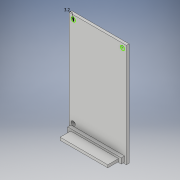
# Autodesk Inventor part: lcd display
Saved by Autodesk Inventor 2017 (Build 210142000, 142)
## iProperties
Created: 2016-11-05
Part Number: lcd display
Material: Generic
Document SubType Name: Modeling
Designer: radrajith
Density: 1 g/cm^3
Appearance: Default
Author: radrajith
Autodesk Inventor part; units mm, degrees
ref_plane "YZ Plane" through (0, 0, 0) normal (1, 0, 0) x (0, 1, 0)
ref_plane "XZ Plane" through (0, 0, 0) normal (0, 1, 0) x (-1, 0, 0)
ref_plane "XY Plane" through (0, 0, 0) normal (0, 0, 1) x (1, 0, 0)
sketch "Sketch1" plane through (0, 0, 0) normal (0, 0, 1) x (1, 0, 0)
  line L0 (42.72, 0) -> (42.72, 77.18)
  line L1 (42.72, 77.18) -> (0, 77.18)
  line L2 (0, 77.18) -> (0, 0)
  line L3 (0, 0) -> (42.72, 0)
  point P0 (0, 0)
  dimension "d0" = 77.18
  dimension "d1" = 42.72
  constraints: 8 end point, 2 parallel, 1 perpendicular
  measures "d0" distance of L2.end L1.end
  measures "d1" distance of L1.end L0.end
extrude "Extrusion1" add sketch "Sketch1" along normal blind 2
sketch "Sketch3" plane through (0, 0, 2) normal (0, 0, 1) x (1, 0, 0)
  line L0 (1.3486, 1.0704) -> (41.3486, 1.0704)
  line L1 (41.3486, 1.0704) -> (41.3486, 5.0704)
  line L2 (41.3486, 5.0704) -> (1.3486, 5.0704)
  line L3 (1.3486, 5.0704) -> (1.3486, 1.0704)
  point P0 (0, 0)
  dimension "d4" = 40
  dimension "d5" = 4
  constraints: 8 end point, 2 parallel, 1 horizontal, 1 perpendicular
  measures "d4" distance of L2.end L1.end
  measures "d5" distance of L1.end L0.end
sketch "Sketch4" plane through (0, 0, 2) normal (0, 0, 1) x (1, 0, 0)
  point P0 (0, 0)
sketch "Sketch5" plane through (0, 0, 2) normal (0, 0, 1) x (1, 0, 0)
  point P0 (0, 0)
extrude "Extrusion2" add sketch "Sketch3" along normal blind 2.54
sketch "Sketch6" plane through (-2.2901, 18.5965, 2) normal (0, 0, 1) x (1, 0, 0)
  line L0 (41.636, -17) -> (41.636, -14.9996)
  line L1 (41.636, -14.9996) -> (6, -14.9996)
  line L2 (6, -14.9996) -> (6, -17)
  line L3 (6, -17) -> (41.636, -17)
  point P0 (0, 0)
  constraints: 8 end point, 2 parallel, 1 perpendicular
extrude "Extrusion3" add sketch "Sketch6" along normal blind 10.54
sketch "Sketch7" plane through (0, 0, 2) normal (0, 0, 1) x (1, 0, 0)
  circle A0 centre (3, 6.92) radius 1.6
  point P0 (0, 0)
  dimension "d11" = 3.2
  constraints: 1 centre point
  measures "d11" diameter of A0
extrude "Extrusion4" cut sketch "Sketch7" against normal blind 2.54
sketch "Sketch8" plane through (0, 0, 2) normal (0, 0, 1) x (1, 0, 0)
  circle A0 centre (3, 74.18) radius 1.6
  circle A1 centre (39.72, 74.18) radius 1.6
  point P0 (0, 0)
  dimension "d14" = 3.2
  constraints: 2 centre point
  measures "d14" diameter of A0
extrude "Extrusion5" cut sketch "Sketch8" against normal blind 2.54
body "Solid1"
